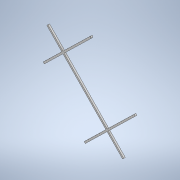
# Autodesk Inventor part: print008_Grundform_Guss_innen
Saved by Autodesk Inventor 2020.3 (Build 243373000, 373)
## iProperties
Created: 2020-03-04
Part Number: print008_Grundform_Guss_innen
Material: Generic
Document SubType Name: Modeling
Designer: Mara
Density: 1 g/cm^3
Appearance: Default
Mass: 1.1982 g
Surface Area: 24.0527 cm^2
Volume: 1.1982 cm^3
Author: Mara
Autodesk Inventor part; units mm, degrees
ref_plane "YZ Plane" through (0, 0, 0) normal (1, 0, 0) x (0, 1, 0)
ref_plane "XZ Plane" through (0, 0, 0) normal (0, 1, 0) x (-1, 0, 0)
ref_plane "XY Plane" through (0, 0, 0) normal (0, 0, 1) x (1, 0, 0)
sketch "Sketch1" plane through (0, 0, 0) normal (0, 0, 1) x (1, 0, 0)
  arc A0 (5.5811, -56.8606) -> (20.209, -64.6836) centre (38.8796, -12.1848) ccw
  arc A1 (-7.6539, -43.4667) -> (5.5811, -56.8606) centre (37.8873, -11.7018) ccw
  arc A2 (-7.6539, -43.4667) -> (-31.2183, -12.0793) centre (-386.265, -303.1724) ccw
  arc A3 (-31.2183, -12.0793) -> (-63.3277, 19.0744) centre (-191.6112, -145.2692) ccw
  arc A4 (-67.5206, 26.3221) -> (-63.3277, 19.0744) centre (-54.6162, 28.9507) ccw
  arc A5 (-66.9469, 41.0059) -> (-67.5206, 26.3221) centre (-15.6776, 31.6496) ccw
  line L0 (-66.9469, 41.0059) -> (-26.0985, 81.0785)
  arc A6 (-3.6955, 79.7027) -> (-26.0985, 81.0785) centre (-17.6076, 36.2535) ccw
  arc A7 (1.4491, 74.6716) -> (-3.6955, 79.7027) centre (-6.1453, 72.0517) ccw
  arc A8 (2.6831, 69.1533) -> (1.4491, 74.6716) centre (-18.5892, 67.2935) ccw
  arc A9 (2.6831, 69.1533) -> (3.1898, 63.5624) centre (229.5421, 86.8959) ccw
  arc A10 (3.1898, 63.5624) -> (8.7161, 49.818) centre (30.4167, 66.5265) ccw
  arc A11 (8.7161, 49.818) -> (19.0471, 39.3259) centre (47.1297, 77.3097) ccw
  arc A12 (19.0471, 39.3259) -> (32.6891, 29.8296) centre (104.4845, 147.5139) ccw
  arc A13 (32.6891, 29.8296) -> (50.5655, 19.6706) centre (502.3948, 835.5524) ccw
  arc A14 (57.8671, 12.5741) -> (50.5655, 19.6706) centre (33.0101, -5.6965) ccw
  arc A15 (67.0572, -4.125) -> (57.8671, 12.5741) centre (18.4686, -19.9867) ccw
  arc A16 (68.9532, -23.0115) -> (67.0572, -4.125) centre (24.8632, -17.8992) ccw
  line L1 (-52.1723, 55.4999) -> (42.0363, -41.3708)
  line L2 (43.4701, -39.9764) -> (-50.7446, 56.9005)
  line L3 (42.0363, -41.3708) -> (43.4701, -39.9764)
  line L4 (-4.2615, -47.8472) -> (57.8671, 12.5741)
  line L5 (56.6239, 14.1548) -> (-5.54, -46.3007)
  line L6 (-55.2456, 12.4327) -> (2.7113, 68.7969)
  line L7 (2.3899, 71.2742) -> (-56.7711, 13.739)
  point P0 (0, 0)
  point P1 (-8.2693, 4.2237)
  point P2 (-4.9861, 4.7501)
  point P3 (-66.0155, 22.3561)
  point P4 (24.203, -20.1649)
  point P5 (22.8086, -18.7311)
  point P6 (-30.7071, 36.2969)
  point P7 (-32.1015, 37.7306)
  point P8 (-33.5353, 36.3363)
  point P9 (-32.1409, 34.9025)
  point P10 (21.3749, -20.1255)
  point P11 (22.7692, -21.5593)
  dimension "d243" = 2
  dimension "d244" = 2
  dimension "d245" = 2
  constraints: 45 point on circle, 17 centre point, 16 end point, 4 parallel, 2 perpendicular, 2 point on line, 2 tangent, 20 other
  measures "d243" distance between parallel lines of L2 L1
  measures "d244" distance between parallel lines of L5 L4
  measures "d245" distance between parallel lines of L7 L6
extrude "Extrusion11" add sketch "Sketch1" along normal blind 2 contours L5 L1 L4 A1 | L5 L2 L4 L1 | L1 L6 L2 L5 | A3 L7 L1 L6 | L4 L2 L3 L1 | L1 L7 L2 L6 | L5 A14 L4 L2 | L1 L0 L2 L7 | L2 L7 A8 A9 L6
body "Solid3"
